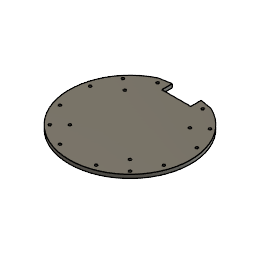
bot (Autodesk Fusion 360 design; units mm, degrees)
Autodesk Fusion 360 part; units mm, degrees
sketch "Esboço1" plane through (0, 0, 0) normal (0, 1, 0) x (1, 0, 0)
  circle A0 centre (0, 0) radius 90
  dimension "d1" = 180
  constraint coincident A0.centre origin
  measures "d1" diameter of A0
sketch "Esboço2" plane through (0, 0, 0) normal (0, 1, 0) x (1, 0, 0)
  circle A0 centre (0, 0) radius 80
  line L0 (0, 0) -> (0, 80)
  line L1 (0, 0) -> (0, -80)
  line L2 (0, 0) -> (80, 0)
  line L3 (0, 0) -> (-80, 0)
  line L4 (0, 0) -> (61.2836, 51.423)
  line L5 (0, 0) -> (80, 0) construction
  line L6 (0, 0) -> (-61.2836, 51.423)
  line L7 (0, 0) -> (80, 0) construction
  line L8 (0, 0) -> (-56.5685, -56.5685)
  line L9 (0, 0) -> (80, 0) construction
  line L10 (0, 0) -> (56.5685, -56.5685)
  line L11 (0, 0) -> (80, 0) construction
  dimension "d2" = 160
  dimension "d3" = 40
  dimension "d4" = 80
  dimension "d5" = 140
  dimension "d6" = 80
  dimension "d7" = 135
  dimension "d8" = 80
  dimension "d9" = 45
  constraint coincident A0.centre L0.start
  constraint coincident A0 L0.end
  constraint vertical L0
  constraint coincident A0 L1.end
  constraint parallel L0 L1
  constraint coincident A0 L2.end
  constraint perpendicular L0 L2
  constraint coincident A0 L3.end
  constraint perpendicular L1 L3
  constraint horizontal L5
  constraint horizontal L7
  constraint horizontal L9
  constraint horizontal L11
  measures "d2" diameter of A0
  measures "d3" angle of L4 L5
  measures "d4" distance of A0.centre L4.end
  measures "d5" angle of L6 L7
  measures "d6" distance of A0.centre L6.end
  measures "d7" angle of L8 L9
  measures "d8" distance of A0.centre L8.end
  measures "d9" angle of L10 L11
sketch "Esboço10" plane through (0, 4, 0) normal (0, 1, 0) x (-1, 0, 0)
  circle A0 centre (0, 0) radius 90
  circle A1 centre (0, 0) radius 80
  dimension "d156" = 160
  constraint coincident A0.centre A1.centre
  measures "d156" diameter of A1
sketch "Esboço11" plane through (0, 4, 0) normal (0, 1, 0) x (-1, 0, 0)
  line L0 (0, 0) -> (0, 89.7923) construction
  line L1 (0, 0) -> (0, -90.4079) construction
  line L2 (0, 0) -> (-89.4844, 0) construction
  line L3 (-89.4844, 0) -> (0, 0) construction
  line L4 (90.1162, 0) -> (0, 0) construction
  line L5 (0, 0) -> (-68.2901, -57.3022) construction
  line L6 (0, 0) -> (180, 0) construction
  line L7 (0, 0) -> (68.944, -57.8509) construction
  line L8 (0, 0) -> (90, 0) construction
  line L9 (0, 0) -> (-63.6396, 63.6396) construction
  line L10 (0, 0) -> (90, 0) construction
  line L11 (0, 0) -> (63.6396, 63.6396) construction
  line L12 (0, 0) -> (90, 0) construction
  dimension "d157" = 140
  dimension "d159" = 40
  dimension "d161" = 135
  dimension "d164" = 45
  constraint coincident L0.start L1.start
  constraint vertical L0
  constraint parallel L0 L1
  constraint perpendicular L0 L2
  constraint perpendicular L1 L4
  constraint horizontal L6
  constraint horizontal L8
  constraint horizontal L10
  constraint horizontal L12
  measures "d157" angle of L5 L6
  measures "d159" angle of L7 L8
  measures "d161" angle of L9 L10
  measures "d164" angle of L11 L12
sketch "Esboço13" plane through (0, 4, 0) normal (0, 1, 0) x (-1, 0, 0)
  line L0 (0, 0) -> (68.944, -57.8509) construction
  line L1 (0, 0) -> (90, 0) construction
  line L2 (68.944, -57.8509) -> (49.7929, -41.7812) construction
  line L3 (62.6595, 0) -> (-0.1598, -74.8652) construction
  line L4 (38.3771, -28.9387) -> (52.197, -12.4687)
  line L5 (35.1632, -32.7689) -> (21.3439, -49.2381)
  line L6 (20.2359, -54.8368) -> (24.0661, -58.0507)
  line L7 (32.9399, -27.6399) -> (34.5469, -25.7248)
  line L8 (32.9399, -27.6399) -> (31.3329, -29.555)
  line L9 (31.3329, -29.555) -> (35.1632, -32.7689)
  line L10 (34.5469, -25.7248) -> (38.3771, -28.9387)
  circle A0 centre (34.855, -29.2468) radius 1.35
  line L11 (50.2508, -38.9019) -> (47.0369, -42.7321)
  line L12 (47.0369, -42.7321) -> (43.2066, -39.5182)
  line L13 (50.2508, -38.9019) -> (46.4206, -35.688)
  circle A1 centre (46.7287, -39.21) radius 1.35
  line L14 (59.4327, -12.0132) -> (57.8257, -13.9283) construction
  circle A2 centre (57.8257, -13.9283) radius 1.35
  line L15 (22.151, -56.4437) -> (23.758, -54.5286) construction
  circle A3 centre (23.758, -54.5286) radius 1.35
  circle A4 centre (0, 0) radius 65 construction
  line L16 (0, 0) -> (0, -90.5075) construction
  line L17 (55.9131, -12.3183) -> (57.5176, -10.4062)
  line L18 (59.7408, -15.5352) -> (61.3478, -13.6201)
  line L19 (55.9131, -12.3183) -> (54.3037, -14.2364)
  line L20 (54.3037, -14.2364) -> (52.197, -12.4687)
  line L21 (58.1339, -17.4503) -> (60.2406, -19.2179)
  line L22 (59.7408, -15.5352) -> (58.1339, -17.4503)
  line L23 (61.3478, -13.6201) -> (57.5176, -10.4062)
  line L24 (27.2801, -54.2205) -> (29.3867, -55.9881)
  line L25 (23.4505, -51.0058) -> (20.2359, -54.8368)
  line L26 (20.2359, -54.8368) -> (24.0661, -58.0507)
  line L27 (24.0661, -58.0507) -> (27.2801, -54.2205)
  line L28 (23.4505, -51.0058) -> (21.3439, -49.2381)
  line L29 (29.3867, -55.9881) -> (43.2066, -39.5182)
  line L30 (46.4206, -35.688) -> (60.2406, -19.2179)
  circle A5 centre (0, 0) radius 53.25 construction
  circle A6 centre (40.7919, -34.2284) radius 7.75 construction
  circle A7 centre (40.7919, -34.2284) radius 26.5 construction
  line L31 (22.151, -56.4437) -> (59.4327, -12.0132) construction
  line L32 (0, 0) -> (0, -90.4079)
  line L33 (-20.2359, -54.8368) -> (-24.0661, -58.0507)
  circle A8 centre (-23.758, -54.5286) radius 1.35
  line L34 (-35.1632, -32.7689) -> (-21.3439, -49.2381)
  line L35 (-31.3329, -29.555) -> (-35.1632, -32.7689)
  line L36 (-32.9399, -27.6399) -> (-31.3329, -29.555)
  line L37 (-32.9399, -27.6399) -> (-34.5469, -25.7248)
  line L38 (-34.5469, -25.7248) -> (-38.3771, -28.9387)
  line L39 (-38.3771, -28.9387) -> (-52.197, -12.4687)
  line L40 (-54.3037, -14.2364) -> (-52.197, -12.4687)
  line L41 (-55.9131, -12.3183) -> (-54.3037, -14.2364)
  line L42 (-55.9131, -12.3183) -> (-57.5176, -10.4062)
  line L43 (-61.3478, -13.6201) -> (-57.5176, -10.4062)
  line L44 (-59.7408, -15.5352) -> (-61.3478, -13.6201)
  line L45 (-59.7408, -15.5352) -> (-58.1339, -17.4503)
  line L46 (-58.1339, -17.4503) -> (-60.2406, -19.2179)
  line L47 (-46.4206, -35.688) -> (-60.2406, -19.2179)
  line L48 (-50.2508, -38.9019) -> (-46.4206, -35.688)
  line L49 (-50.2508, -38.9019) -> (-47.0369, -42.7321)
  line L50 (-47.0369, -42.7321) -> (-43.2066, -39.5182)
  line L51 (-29.3867, -55.9881) -> (-43.2066, -39.5182)
  line L52 (-27.2801, -54.2205) -> (-29.3867, -55.9881)
  line L53 (-23.4505, -51.0058) -> (-21.3439, -49.2381)
  circle A9 centre (-46.7287, -39.21) radius 1.35
  circle A10 centre (-34.855, -29.2468) radius 1.35
  circle A11 centre (-57.8257, -13.9283) radius 1.35
  line L54 (-24.0661, -58.0507) -> (-27.2801, -54.2205)
  line L55 (-23.4505, -51.0058) -> (-20.2359, -54.8368)
  line L56 (50.2508, -38.9019) -> (47.0369, -42.7321)
  line L57 (47.0369, -42.7321) -> (43.2066, -39.5182)
  circle A12 centre (46.7287, -39.21) radius 1.35
  line L58 (50.2508, -38.9019) -> (46.4206, -35.688)
  line L59 (46.4206, -35.688) -> (60.2406, -19.2179)
  line L60 (59.7408, -15.5352) -> (58.1339, -17.4503)
  circle A13 centre (57.8257, -13.9283) radius 1.35
  line L61 (58.1339, -17.4503) -> (60.2406, -19.2179)
  line L62 (59.7408, -15.5352) -> (61.3478, -13.6201)
  line L63 (61.3478, -13.6201) -> (57.5176, -10.4062)
  line L64 (55.9131, -12.3183) -> (54.3037, -14.2364)
  line L65 (55.9131, -12.3183) -> (57.5176, -10.4062)
  line L66 (54.3037, -14.2364) -> (52.197, -12.4687)
  line L67 (38.3771, -28.9387) -> (52.197, -12.4687)
  line L68 (34.5469, -25.7248) -> (38.3771, -28.9387)
  circle A14 centre (34.855, -29.2468) radius 1.35
  line L69 (31.3329, -29.555) -> (35.1632, -32.7689)
  line L70 (32.9399, -27.6399) -> (34.5469, -25.7248)
  line L71 (32.9399, -27.6399) -> (31.3329, -29.555)
  line L72 (35.1632, -32.7689) -> (21.3439, -49.2381)
  line L73 (29.3867, -55.9881) -> (43.2066, -39.5182)
  line L74 (27.2801, -54.2205) -> (29.3867, -55.9881)
  line L75 (24.0661, -58.0507) -> (27.2801, -54.2205)
  line L76 (20.2359, -54.8368) -> (24.0661, -58.0507)
  circle A15 centre (23.758, -54.5286) radius 1.35
  line L77 (23.4505, -51.0058) -> (20.2359, -54.8368)
  line L78 (23.4505, -51.0058) -> (21.3439, -49.2381)
  line L79 (0, 0) -> (63.6396, 63.6396) construction
  line L80 (0, 0) -> (90, 0) construction
  line L81 (63.6396, 63.6396) -> (33.9411, 33.9411) construction
  line L82 (33.9411, 33.9411) -> (0, 67.8823) construction
  line L83 (33.9411, 33.9411) -> (67.8823, 0) construction
  line L84 (0, 0) -> (0, 90) construction
  line L85 (0, 0) -> (-89.8338, 0) construction
  line L86 (41.7925, 40.6545) -> (26.5896, 55.8573)
  line L87 (24.6452, 53.9127) -> (26.5896, 55.8573)
  line L88 (22.8773, 55.6805) -> (24.6452, 53.9127)
  line L89 (22.8773, 55.6805) -> (21.1096, 57.4483)
  line L90 (21.1096, 57.4483) -> (17.5741, 53.9127)
  line L91 (19.3391, 52.1477) -> (17.5741, 53.9127)
  line L92 (19.3391, 52.1477) -> (21.1096, 50.3772)
  circle A16 centre (21.1096, 53.9127) radius 1.35
  line L93 (21.1096, 50.3772) -> (19.1651, 48.4327)
  line L94 (34.3679, 33.2299) -> (19.1651, 48.4327)
  line L95 (30.8323, 29.6943) -> (34.3679, 33.2299)
  circle A17 centre (34.3679, 29.6943) radius 1.35
  line L96 (32.6001, 27.9266) -> (30.8323, 29.6943)
  line L97 (32.6001, 27.9266) -> (34.3679, 26.1588)
  line L98 (34.3679, 26.1588) -> (37.9034, 29.6943)
  line L99 (37.9034, 29.6943) -> (53.1055, 14.4923)
  line L100 (45.328, 44.19) -> (41.7925, 40.6545)
  line L101 (45.328, 44.19) -> (48.8636, 40.6545)
  line L102 (48.8636, 40.6545) -> (45.328, 37.119)
  circle A18 centre (45.328, 40.6545) radius 1.35
  line L103 (60.5308, 21.9162) -> (45.328, 37.119)
  line L104 (62.1218, 16.4361) -> (58.5863, 19.9716)
  line L105 (58.5863, 19.9716) -> (60.5308, 21.9162)
  line L106 (55.05, 16.4368) -> (58.5863, 12.9005)
  line L107 (55.05, 16.4368) -> (53.1055, 14.4923)
  line L108 (58.5863, 12.9005) -> (62.1218, 16.4361)
  circle A19 centre (58.5863, 16.4361) radius 1.35
  line L109 (-58.5863, 12.9005) -> (-62.1218, 16.4361)
  line L110 (-55.05, 16.4368) -> (-58.5863, 12.9005)
  circle A20 centre (-58.5863, 16.4361) radius 1.35
  line L111 (-62.1218, 16.4361) -> (-58.5863, 19.9716)
  line L112 (-58.5863, 19.9716) -> (-60.5308, 21.9162)
  line L113 (-55.05, 16.4368) -> (-53.1055, 14.4923)
  line L114 (-37.9034, 29.6943) -> (-53.1055, 14.4923)
  line L115 (-60.5308, 21.9162) -> (-45.328, 37.119)
  line L116 (-48.8636, 40.6545) -> (-45.328, 37.119)
  line L117 (-45.328, 44.19) -> (-48.8636, 40.6545)
  circle A21 centre (-45.328, 40.6545) radius 1.35
  line L118 (-45.328, 44.19) -> (-41.7925, 40.6545)
  line L119 (-41.7925, 40.6545) -> (-26.5896, 55.8573)
  line L120 (-34.3679, 26.1588) -> (-37.9034, 29.6943)
  line L121 (-32.6001, 27.9266) -> (-34.3679, 26.1588)
  line L122 (-32.6001, 27.9266) -> (-30.8323, 29.6943)
  circle A22 centre (-34.3679, 29.6943) radius 1.35
  line L123 (-30.8323, 29.6943) -> (-34.3679, 33.2299)
  line L124 (-34.3679, 33.2299) -> (-19.1651, 48.4327)
  line L125 (-24.6452, 53.9127) -> (-26.5896, 55.8573)
  line L126 (-22.8773, 55.6805) -> (-24.6452, 53.9127)
  line L127 (-22.8773, 55.6805) -> (-21.1096, 57.4483)
  circle A23 centre (-21.1096, 53.9127) radius 1.35
  line L128 (-21.1096, 57.4483) -> (-17.5741, 53.9127)
  line L129 (-19.3391, 52.1477) -> (-17.5741, 53.9127)
  line L130 (-19.3391, 52.1477) -> (-21.1096, 50.3772)
  line L131 (-21.1096, 50.3772) -> (-19.1651, 48.4327)
  line L132 (0, -65) -> (15, -65)
  line L133 (0, -65) -> (-15, -65)
  line L134 (-15, -65) -> (-15, -55)
  line L135 (-15, -55) -> (15, -55)
  line L136 (15, -55) -> (15, -65)
  line L137 (15, -65) -> (15, -80)
  line L138 (15, -80) -> (-15, -80)
  line L139 (-15, -80) -> (-15, -65)
  dimension "d166" = 40
  dimension "d167" = 25
  dimension "d176" = 2.5
  dimension "d177" = 2.5
  dimension "d178" = 5
  dimension "d179" = 2.7
  dimension "d182" = 5
  dimension "d183" = 2.7
  dimension "d186" = 2.7
  dimension "d187" = 2.5
  dimension "d188" = 2.7
  dimension "d194" = 5
  dimension "d195" = 2.5
  dimension "d196" = 2.75
  dimension "d197" = 2.75
  dimension "d199" = 13.5118
  dimension "d200" = 15.0096
  dimension "d201" = 21.5
  dimension "d202" = 21.499
  dimension "d203" = 2.5
  dimension "d204" = 2.5
  dimension "d205" = 2.5
  dimension "d206" = 2.5
  dimension "d207" = 5
  dimension "d208" = 2.75
  dimension "d209" = 2.75
  dimension "d210" = 5
  dimension "d211" = 5
  dimension "d212" = 5
  dimension "d215" = 29
  dimension "d216" = 24.1299
  dimension "d217" = 24.1299
  dimension "d218" = 2.5
  dimension "d220" = 2.5
  dimension "d222" = 2.5
  dimension "d223" = 2.5
  dimension "d224" = 2.5
  dimension "d225" = 5
  dimension "d226" = 2.7
  dimension "d227" = 5
  dimension "d228" = 2.7
  dimension "d229" = 2.7
  dimension "d230" = 2.7
  dimension "d231" = 5
  dimension "d232" = 2.5
  dimension "d233" = 2.75
  dimension "d234" = 2.75
  dimension "d235" = 21.5
  dimension "d236" = 21.499
  dimension "d237" = 2.5
  dimension "d238" = 2.5
  dimension "d239" = 2.5
  dimension "d240" = 2.5
  dimension "d241" = 5
  dimension "d242" = 2.75
  dimension "d243" = 2.75
  dimension "d244" = 5
  dimension "d245" = 5
  dimension "d246" = 5
  dimension "d247" = 2.5
  dimension "d248" = 2.5
  dimension "d249" = 45
  dimension "d250" = 90
  dimension "d251" = 42
  dimension "d252" = 90
  dimension "d253" = 5
  dimension "d254" = 2.7
  dimension "d255" = 5
  dimension "d256" = 2.7
  dimension "d257" = 2.7
  dimension "d258" = 5
  dimension "d259" = 2.75
  dimension "d260" = 2.75
  dimension "d261" = 21.5
  dimension "d262" = 21.499
  dimension "d263" = 2.5
  dimension "d264" = 2.5
  dimension "d265" = 5
  dimension "d266" = 2.75
  dimension "d267" = 5
  dimension "d268" = 5
  dimension "d269" = 2.5
  dimension "d270" = 2.5
  dimension "d271" = 2.5
  dimension "d272" = 2.7
  dimension "d273" = 21.499
  dimension "d274" = 2.75
  dimension "d275" = 2.5
  dimension "d283" = 15
  dimension "d284" = 15
  dimension "d285" = 10
  dimension "d286" = 30
  dimension "d287" = 15
  dimension "d288" = 30
  constraint horizontal L1
  constraint coincident L0.start L1.start
  constraint parallel L0 L2
  constraint coincident L1 L3.start
  constraint perpendicular L0 L3
  constraint perpendicular L0 L4
  constraint perpendicular L3 L6
  constraint perpendicular L0 L7
  constraint perpendicular L0 L8
  constraint coincident L3 L5.start
  constraint perpendicular L8 L9
  constraint perpendicular L4 L10
  constraint coincident L14.end A2.centre
  constraint perpendicular L6 L15
  constraint coincident L15.end A3.centre
  constraint coincident L2.end A4
  constraint vertical L16
  constraint perpendicular L21 L22
  constraint parallel L17 L19
  constraint parallel L3 L19
  constraint coincident L3 L5.end
  constraint perpendicular L6 L25
  constraint perpendicular L15 L26
  constraint perpendicular L24 L27
  constraint coincident L6 L15.start
  constraint collinear L29 L30
  constraint perpendicular L11 L12
  constraint coincident L0 A6.centre
  constraint coincident A5 A6.centre
  constraint coincident A0.centre A6
  constraint concentric A6 A7
  constraint coincident L15.end A7
  constraint parallel L6 L28
  constraint parallel L24 L26
  constraint perpendicular L23 L31
  constraint parallel L25 L31
  constraint parallel L11 L31
  constraint perpendicular L13 L30
  constraint perpendicular L12 L29
  constraint perpendicular L19 L20
  constraint symmetric L7.start L32 L36.start
  constraint symmetric L7.end L32 L37.end
  constraint symmetric L8.end L32 L35.start
  constraint symmetric L5.start L32 L34.start
  constraint symmetric L4.start L32 L38.end
  constraint symmetric A0 L32 A10
  constraint symmetric L11.start L32 L48.start
  constraint symmetric L11.end L32 L49.end
  constraint symmetric L12.end L32 L50.end
  constraint symmetric L13.end L32 L47.start
  constraint symmetric A1 L32 A9
  constraint symmetric A2 L32 A11
  constraint symmetric A3 L32 A8
  constraint symmetric L18.start L32 L44.start
  constraint symmetric L17.start L32 L41.start
  constraint symmetric L17.end L32 L42.end
  constraint symmetric L18.end L32 L43.start
  constraint symmetric L19.end L32 L40.start
  constraint symmetric L4.end L32 L39.end
  constraint symmetric L21.end L32 L46.end
  constraint symmetric L21.start L32 L45.end
  constraint symmetric L5.end L32 L34.end
  constraint symmetric L24.end L32 L51.start
  constraint symmetric L25.start L32 L53.start
  constraint symmetric L6.start L32 L33.start
  constraint symmetric L6.end L32 L33.end
  constraint symmetric L24.start L32 L52.start
  constraint perpendicular L69 L71
  constraint perpendicular L67 L68
  constraint perpendicular L60 L61
  constraint parallel L64 L65
  constraint perpendicular L76 L77
  constraint perpendicular L74 L75
  constraint collinear L59 L73
  constraint perpendicular L56 L57
  constraint parallel L76 L78
  constraint perpendicular L58 L59
  constraint perpendicular L57 L73
  constraint perpendicular L64 L66
  constraint horizontal L80
  constraint parallel L79 L81
  constraint perpendicular L79 L82
  constraint coincident L1 L83.end
  constraint perpendicular L81 L83
  constraint vertical L84
  constraint coincident L84 L82.end
  constraint parallel L1 L85
  constraint perpendicular L94 L95
  constraint perpendicular L87 L88
  constraint perpendicular L106 L108
  constraint perpendicular L104 L105
  constraint parallel L107 L108
  constraint perpendicular L92 L93
  constraint symmetric L84 L91.start L129.start
  constraint symmetric L84 L89.end L127.end
  constraint symmetric L84 L93.end L124.end
  constraint symmetric L84 L86.end L119.end
  constraint symmetric L84 L88.start L126.start
  constraint symmetric L84 L92.end L130.end
  constraint symmetric L84 L97.end L120.start
  constraint symmetric L84 L99.end L113.end
  constraint symmetric L84 L95.start L122.end
  constraint symmetric L84 L98.end L114.start
  constraint symmetric L84 L94.start L123.end
  constraint symmetric L84 L90.end L128.end
  constraint symmetric L84 L101.end L116.start
  constraint symmetric L84 L100.start L117.start
  constraint symmetric L84 L102.end L115.end
  constraint symmetric L84 L86.start L118.end
  constraint symmetric L84 L104.start L109.end
  constraint symmetric L84 L87.start L125.start
  constraint symmetric L84 L104.end L111.end
  constraint symmetric L84 L103.start L112.end
  constraint symmetric L84 L106.start L110.start
  constraint symmetric L84 L106.end L109.start
  constraint symmetric L84 L96.start L121.start
  constraint symmetric L84 A16 A23
  constraint symmetric L84 A17 A22
  constraint symmetric L84 A18 A21
  constraint symmetric L84 A19 A20
  constraint coincident L32 L132.start
  constraint coincident A4 L132.start
  constraint perpendicular L32 L132
  constraint perpendicular L16 L133
  constraint perpendicular L133 L134
  constraint perpendicular L134 L135
  constraint perpendicular L132 L137
  constraint perpendicular L32 L138
  measures "d166" angle of L0 L1
  measures "d167" distance of L0.end L2.end
  measures "d176" distance of L7.start L7.end
  measures "d177" distance of L7.start L8.end
  measures "d178" distance of L7.end L4.start
  measures "d179" diameter of A0
  measures "d182" distance of L11.start L11.end
  measures "d183" diameter of A1
  measures "d186" diameter of A2
  measures "d187" distance of L15.start L15.end
  measures "d188" diameter of A3
  measures "d194" distance of L6.start L6.end
  measures "d195" distance of L15.end L25
  measures "d196" distance of L5.end L25.start
  measures "d197" distance of L24.end L24.start
  measures "d199" horizontal distance of L24.start A6.centre
  measures "d200" vertical distance of L5.end A6.centre
  measures "d201" distance of L12.end L24.end
  measures "d202" distance of L5.start L5.end
  measures "d203" distance of L7.start A0.centre
  measures "d204" distance of L9 A0.centre
  measures "d205" distance of L12 A1.centre
  measures "d206" distance of L11 A1.centre
  measures "d207" distance of L11.start L13.end
  measures "d208" distance of L21.end L21.start
  measures "d209" distance of L19.end L4.end
  measures "d210" distance of L17.end L19.end
  measures "d211" distance of L17.end L18.end
  measures "d212" distance of L18.end L21.start
  measures "d215" distance of L14.start A6.centre
  measures "d216" distance of L19.end A6.centre
  measures "d217" distance of L21.start A6.centre
  measures "d218" distance of L14.start L14.end
  measures "d220" distance of L18.start L18.end
  measures "d222" distance of L14.end L19
  measures "d223" distance of L7.start L7.end
  measures "d224" distance of L7.start L8.end
  measures "d225" distance of L7.end L4.start
  measures "d226" diameter of A14
  measures "d227" distance of L11.end L11.start
  measures "d228" diameter of A12
  measures "d229" diameter of A13
  measures "d230" diameter of A15
  measures "d231" distance of L6.end L6.start
  measures "d232" distance of L15.end L77
  measures "d233" distance of L5.end L25.start
  measures "d234" distance of L24.start L24.end
  measures "d235" distance of L12.end L24.end
  measures "d236" distance of L5.end L5.start
  measures "d237" distance of L7.start A0.centre
  measures "d238" distance of A0.centre L69
  measures "d239" distance of A1.centre L57
  measures "d240" distance of A1.centre L56
  measures "d241" distance of L11.start L13.end
  measures "d242" distance of L21.start L21.end
  measures "d243" distance of L4.end L19.end
  measures "d244" distance of L17.end L19.end
  measures "d245" distance of L17.end L18.end
  measures "d246" distance of L21.start L18.end
  measures "d247" distance of L18.start L18.end
  measures "d248" distance of L14.end L64
  measures "d249" angle of L79 L80
  measures "d250" distance of L0.start L79.end
  measures "d251" distance of L79.end L81.end
  measures "d252" distance of L0.start L84.end
  measures "d253" distance of L95.start L94.start
  measures "d254" diameter of A17
  measures "d255" distance of L101.end L100.start
  measures "d256" diameter of A18
  measures "d257" diameter of A16
  measures "d258" distance of L104.start L106.end
  measures "d259" distance of L99.end L106.start
  measures "d260" distance of L104.end L103.start
  measures "d261" distance of L102.end L103.start
  measures "d262" distance of L99.end L98.end
  measures "d263" distance of A17.centre L98
  measures "d264" distance of A18.centre L101
  measures "d265" distance of L100.start L86.start
  measures "d266" distance of L87.start L86.end
  measures "d267" distance of L90.end L89.end
  measures "d268" distance of L87.start L89.end
  measures "d269" distance of L88.start L89.end
  measures "d270" distance of L96.start L95.start
  measures "d271" distance of L96.start L97.end
  measures "d272" diameter of A19
  measures "d273" distance of L99.end L98.end
  measures "d274" distance of L93.end L92.end
  measures "d275" distance of L89.end L88.start
  measures "d283" distance of L132.start L132.end
  measures "d284" distance of L132.start L133.end
  measures "d285" distance of L133.end L134.end
  measures "d286" distance of L134.end L135.end
  measures "d287" distance of L132.end L137.end
  measures "d288" distance of L137.end L138.end
sketch "Esboço14" plane through (0, 4, 0) normal (0, 1, 0) x (-1, 0, 0)
  circle A0 centre (0, 0) radius 90
  circle A1 centre (0, 0) radius 67.5
  dimension "d276" = 135
  constraint coincident A0.centre A1.centre
  measures "d276" diameter of A1
sketch "Esboço15" plane through (0, 0, 0) normal (0, 1, 0) x (1, 0, 0)
  line L0 (0, 0) -> (0, 92.4179) construction
  line L1 (0, 0) -> (93.6244, 0) construction
  line L2 (0, 0) -> (0, -88.0745) construction
  line L3 (0, 0) -> (-79.8703, 0) construction
  line L4 (0, 0) -> (88.3333, 0) construction
  line L5 (0, 0) -> (-68.7403, 57.6799) construction
  line L6 (0, 0) -> (89.7341, 0) construction
  line L7 (0, 0) -> (60.1115, -60.1115) construction
  line L8 (0, 0) -> (85.0106, 0) construction
  line L9 (0, 0) -> (-55.023, -55.023) construction
  line L10 (0, 0) -> (77.8143, 0) construction
  line L11 (0, 0) -> (-42.1324, 35.3533) construction
  line L12 (0, 0) -> (-38.8909, -38.8909) construction
  line L13 (-42.1324, 35.3533) -> (-35.7046, 43.0138) construction
  line L14 (-42.1324, 35.3533) -> (-48.5603, 27.6929) construction
  line L15 (-38.8909, -38.8909) -> (-45.9619, -31.8198) construction
  line L16 (-38.8909, -38.8909) -> (-31.8198, -45.9619) construction
  line L17 (-36.2801, 33.7714) -> (-22.428, 50.2797)
  line L18 (-53.4104, 13.3563) -> (-39.5583, 29.8646)
  line L19 (-50.3291, 42.2311) -> (-48.69, 44.1846)
  line L20 (-50.3291, 42.2311) -> (-51.9682, 40.2777)
  line L21 (-51.9682, 40.2777) -> (-48.0614, 36.9995)
  line L22 (-48.69, 44.1846) -> (-44.7832, 40.9063)
  line L23 (-30.9311, 57.4146) -> (-44.7832, 40.9063)
  line L24 (-48.0614, 36.9995) -> (-61.9135, 20.4913)
  line L25 (-23.4013, 57.754) -> (-21.4479, 56.1148)
  line L26 (-23.4013, 57.754) -> (-25.3548, 59.3931)
  line L27 (-21.4479, 56.1148) -> (-24.7262, 52.208)
  line L28 (-25.3548, 59.3931) -> (-28.633, 55.4862)
  line L29 (-22.428, 50.2797) -> (-24.7262, 52.208)
  line L30 (-28.633, 55.4862) -> (-30.9311, 57.4146)
  line L31 (-60.9401, 13.017) -> (-62.8936, 14.6561)
  line L32 (-60.9401, 13.017) -> (-58.9867, 11.3779)
  line L33 (-58.9867, 11.3779) -> (-55.7085, 15.2847)
  line L34 (-62.8936, 14.6561) -> (-59.6153, 18.5629)
  line L35 (-61.9135, 20.4913) -> (-59.6153, 18.5629)
  line L36 (-55.7085, 15.2847) -> (-53.4104, 13.3563)
  line L37 (-60.9401, 13.017) -> (-23.4013, 57.754) construction
  line L38 (-39.5583, 29.8646) -> (-36.0345, 26.9078)
  line L39 (-36.2801, 33.7714) -> (-32.7563, 30.8146)
  line L40 (-36.0345, 26.9078) -> (-32.7563, 30.8146)
  line L41 (-36.7696, -33.1633) -> (-52.0077, -17.9252)
  line L42 (-33.1633, -36.7696) -> (-17.9252, -52.0077)
  line L43 (-31.7137, -31.7137) -> (-29.9106, -33.5169)
  line L44 (-31.7137, -31.7137) -> (-33.5169, -29.9106)
  line L45 (-29.9106, -33.5169) -> (-33.1633, -36.7696)
  line L46 (-33.5169, -29.9106) -> (-36.7696, -33.1633)
  line L47 (-18.2434, -59.5384) -> (-16.4402, -57.7353)
  line L48 (-18.2434, -59.5384) -> (-20.0465, -61.3415)
  line L49 (-20.0465, -61.3415) -> (-23.6527, -57.7353)
  line L50 (-16.4402, -57.7353) -> (-20.0465, -54.129)
  line L51 (-59.5384, -18.2434) -> (-57.7353, -16.4402)
  line L52 (-59.5384, -18.2434) -> (-61.3415, -20.0465)
  line L53 (-61.3415, -20.0465) -> (-57.7353, -23.6527)
  line L54 (-57.7353, -16.4402) -> (-54.129, -20.0465)
  line L55 (-46.4216, -46.4216) -> (-44.6184, -48.2247)
  line L56 (-46.4216, -46.4216) -> (-48.2247, -44.6184)
  line L57 (-48.2247, -44.6184) -> (-44.6184, -41.0122)
  line L58 (-44.6184, -48.2247) -> (-41.0122, -44.6184)
  line L59 (-59.8566, -25.774) -> (-57.7353, -23.6527)
  line L60 (-54.129, -20.0465) -> (-52.0077, -17.9252)
  line L61 (-25.774, -59.8566) -> (-41.0122, -44.6184)
  line L62 (-44.6184, -41.0122) -> (-59.8566, -25.774)
  line L63 (-17.9252, -52.0077) -> (-20.0465, -54.129)
  line L64 (-23.6527, -57.7353) -> (-25.774, -59.8566)
  circle A0 centre (-57.6999, -20.0818) radius 1.4
  circle A1 centre (-33.3754, -33.3754) radius 1.4
  circle A2 centre (-44.5831, -44.5831) radius 1.4
  circle A3 centre (-20.0818, -57.6999) radius 1.4
  circle A4 centre (-36.1956, 30.3717) radius 1.4
  circle A5 centre (-48.3374, 40.5599) radius 1.4
  circle A6 centre (-25.0726, 55.7622) radius 1.4
  circle A7 centre (-59.2689, 15.0087) radius 1.4
  line L65 (50.3291, 42.2311) -> (51.9682, 40.2777)
  circle A8 centre (48.3374, 40.5599) radius 1.4
  line L66 (28.633, 55.4862) -> (30.9311, 57.4146)
  line L67 (25.3548, 59.3931) -> (28.633, 55.4862)
  line L68 (42.1324, 35.3533) -> (35.7046, 43.0138) construction
  line L69 (58.9867, 11.3779) -> (55.7085, 15.2847)
  line L70 (60.9401, 13.017) -> (62.8936, 14.6561)
  line L71 (55.7085, 15.2847) -> (53.4104, 13.3563)
  line L72 (53.4104, 13.3563) -> (39.5583, 29.8646)
  line L73 (39.5583, 29.8646) -> (36.0345, 26.9078)
  line L74 (62.8936, 14.6561) -> (59.6153, 18.5629)
  line L75 (22.428, 50.2797) -> (24.7262, 52.208)
  line L76 (23.4013, 57.754) -> (21.4479, 56.1148)
  line L77 (50.3291, 42.2311) -> (48.69, 44.1846)
  line L78 (60.9401, 13.017) -> (23.4013, 57.754) construction
  line L79 (21.4479, 56.1148) -> (24.7262, 52.208)
  line L80 (42.1324, 35.3533) -> (48.5603, 27.6929) construction
  line L81 (36.0345, 26.9078) -> (32.7563, 30.8146)
  line L82 (36.2801, 33.7714) -> (22.428, 50.2797)
  line L83 (60.9401, 13.017) -> (58.9867, 11.3779)
  circle A9 centre (59.2689, 15.0087) radius 1.4
  line L84 (30.9311, 57.4146) -> (44.7832, 40.9063)
  line L85 (48.0614, 36.9995) -> (61.9135, 20.4913)
  line L86 (48.69, 44.1846) -> (44.7832, 40.9063)
  line L87 (61.9135, 20.4913) -> (59.6153, 18.5629)
  line L88 (23.4013, 57.754) -> (25.3548, 59.3931)
  line L89 (51.9682, 40.2777) -> (48.0614, 36.9995)
  circle A10 centre (36.1956, 30.3717) radius 1.4
  circle A11 centre (25.0726, 55.7622) radius 1.4
  line L90 (36.2801, 33.7714) -> (32.7563, 30.8146)
  line L91 (18.2434, -59.5384) -> (20.0465, -61.3415)
  line L92 (16.4402, -57.7353) -> (20.0465, -54.129)
  line L93 (23.6527, -57.7353) -> (25.774, -59.8566)
  line L94 (17.9252, -52.0077) -> (20.0465, -54.129)
  line L95 (54.129, -20.0465) -> (52.0077, -17.9252)
  line L96 (48.2247, -44.6184) -> (44.6184, -41.0122)
  circle A12 centre (57.6999, -20.0818) radius 1.4
  line L97 (44.6184, -48.2247) -> (41.0122, -44.6184)
  line L98 (61.3415, -20.0465) -> (57.7353, -23.6527)
  line L99 (38.8909, -38.8909) -> (31.8198, -45.9619) construction
  line L100 (59.5384, -18.2434) -> (61.3415, -20.0465)
  line L101 (57.7353, -16.4402) -> (54.129, -20.0465)
  line L102 (31.7137, -31.7137) -> (29.9106, -33.5169)
  line L103 (31.7137, -31.7137) -> (33.5169, -29.9106)
  line L104 (38.8909, -38.8909) -> (45.9619, -31.8198) construction
  circle A13 centre (33.3754, -33.3754) radius 1.4
  line L105 (46.4216, -46.4216) -> (44.6184, -48.2247)
  line L106 (59.8566, -25.774) -> (57.7353, -23.6527)
  line L107 (0, 0) -> (38.8909, -38.8909) construction
  line L108 (46.4216, -46.4216) -> (48.2247, -44.6184)
  circle A14 centre (44.5831, -44.5831) radius 1.4
  line L109 (20.0465, -61.3415) -> (23.6527, -57.7353)
  circle A15 centre (20.0818, -57.6999) radius 1.4
  line L110 (0, 0) -> (55.023, -55.023) construction
  line L111 (44.6184, -41.0122) -> (59.8566, -25.774)
  line L112 (59.5384, -18.2434) -> (57.7353, -16.4402)
  line L113 (25.774, -59.8566) -> (41.0122, -44.6184)
  line L114 (18.2434, -59.5384) -> (16.4402, -57.7353)
  line L115 (36.7696, -33.1633) -> (52.0077, -17.9252)
  line L116 (33.5169, -29.9106) -> (36.7696, -33.1633)
  line L117 (29.9106, -33.5169) -> (33.1633, -36.7696)
  line L118 (33.1633, -36.7696) -> (17.9252, -52.0077)
  point P0 (68.7403, 57.6799)
  dimension "d294" = 45
  dimension "d295" = 135
  dimension "d296" = 55
  dimension "d297" = 55
  dimension "d298" = 10
  dimension "d299" = 10
  dimension "d300" = 10
  dimension "d301" = 10
  dimension "d305" = 11.1
  dimension "d306" = 48.2
  dimension "d307" = 11.1
  dimension "d318" = 2.55
  dimension "d319" = 2.55
  dimension "d321" = 2.55
  dimension "d322" = 2.55
  dimension "d324" = 2.55
  dimension "d325" = 2.55
  dimension "d328" = 4.6
  dimension "d333" = 11.1
  dimension "d334" = 48.2
  dimension "d336" = 2.55
  dimension "d337" = 2.55
  dimension "d340" = 2.55
  dimension "d341" = 2.55
  dimension "d344" = 2.55
  dimension "d345" = 2.55
  dimension "d348" = 2.55
  dimension "d349" = 2.55
  dimension "d365" = 2.8
  dimension "d367" = 2.8
  dimension "d369" = 2.8
  dimension "d371" = 2.8
  dimension "d373" = 2.8
  dimension "d375" = 2.8
  dimension "d377" = 2.8
  dimension "d379" = 2.8
  constraint coincident L0.start L1.start
  constraint vertical L0
  constraint perpendicular L0 L1
  constraint perpendicular L1 L2
  constraint perpendicular L2 L3
  constraint horizontal L4
  constraint horizontal L6
  constraint horizontal L8
  constraint horizontal L10
  constraint parallel L5 L11
  constraint parallel L9 L12
  constraint perpendicular L5 L13
  constraint perpendicular L5 L14
  constraint perpendicular L9 L15
  constraint perpendicular L9 L16
  constraint perpendicular L5 L17
  constraint perpendicular L17 L29
  constraint perpendicular L5 L23
  constraint perpendicular L23 L35
  constraint perpendicular L5 L19
  constraint perpendicular L21 L23
  constraint perpendicular L22 L23
  constraint coincident L21.end L23
  constraint collinear L23 L24
  constraint perpendicular L27 L29
  constraint coincident L28.end L29
  constraint perpendicular L28 L29
  constraint collinear L29 L30
  constraint coincident L33.end L35
  constraint perpendicular L33 L35
  constraint perpendicular L34 L35
  constraint collinear L35 L36
  constraint perpendicular L25 L37
  constraint perpendicular L17 L39
  constraint perpendicular L39 L40
  constraint perpendicular L12 L41
  constraint perpendicular L12 L42
  constraint perpendicular L42 L63
  constraint perpendicular L9 L61
  constraint perpendicular L9 L43
  constraint perpendicular L12 L44
  constraint perpendicular L42 L45
  constraint perpendicular L41 L46
  constraint coincident L49.end L63
  constraint perpendicular L49 L63
  constraint perpendicular L50 L63
  constraint perpendicular L53 L59
  constraint perpendicular L54 L59
  constraint coincident L54.end L59
  constraint perpendicular L9 L55
  constraint coincident L57.end L61
  constraint perpendicular L57 L61
  constraint perpendicular L58 L61
  constraint collinear L59 L60
  constraint collinear L61 L62
  constraint collinear L63 L64
  constraint symmetric L0 L5.end P0
  constraint symmetric L0 L11.end L68.start
  constraint symmetric L0 L13.end L68.end
  constraint symmetric L0 L14.end L80.end
  constraint symmetric L0 L17.end L75.start
  constraint symmetric L0 L23.start L66.end
  constraint symmetric L0 L24.end L85.end
  constraint symmetric L0 L18.start L71.end
  constraint symmetric L0 L19.start L65.start
  constraint symmetric L0 L25.start L76.start
  constraint symmetric L0 L31.start L70.start
  constraint symmetric L0 L17.start L82.start
  constraint symmetric L0 L18.end L72.end
  constraint symmetric L0 L19.end L77.end
  constraint symmetric L0 L20.end L65.end
  constraint symmetric L0 L22.end L84.end
  constraint symmetric L0 L21.end L85.start
  constraint symmetric L0 L25.end L76.end
  constraint symmetric L0 L26.end L67.start
  constraint symmetric L0 L27.end L75.end
  constraint symmetric L0 L28.end L66.start
  constraint symmetric L0 L31.end L70.end
  constraint symmetric L0 L32.end L69.start
  constraint symmetric L0 L33.end L69.end
  constraint symmetric L0 L34.end L74.end
  constraint symmetric L0 L38.end L73.end
  constraint symmetric L0 L39.end L81.end
  constraint symmetric L0 A4 A10
  constraint symmetric L0 A5 A8
  constraint symmetric L0 A6 A11
  constraint symmetric L0 A7 A9
  constraint symmetric L2 L0.start L1.start
  constraint symmetric L2 L9.end L110.end
  constraint symmetric L2 L12.end L99.start
  constraint symmetric L2 L15.end L104.end
  constraint symmetric L2 L16.end L99.end
  constraint symmetric L2 L41.end L95.end
  constraint symmetric L2 L42.end L94.start
  constraint symmetric L2 L61.start L93.end
  constraint symmetric L2 L59.start L106.start
  constraint symmetric L2 L43.start L102.start
  constraint symmetric L2 L43.end L102.end
  constraint symmetric L2 L44.end L103.end
  constraint symmetric L2 L42.start L117.end
  constraint symmetric L2 L41.start L115.start
  constraint symmetric L2 L47.start L91.start
  constraint symmetric L2 L47.end L92.start
  constraint symmetric L2 L48.end L91.end
  constraint symmetric L2 L49.end L93.start
  constraint symmetric L2 L50.end L92.end
  constraint symmetric L2 L51.start L100.start
  constraint symmetric L2 L51.end L101.start
  constraint symmetric L2 L52.end L98.start
  constraint symmetric L2 L53.end L98.end
  constraint symmetric L2 L54.end L95.start
  constraint symmetric L2 L55.start L105.start
  constraint symmetric L2 L55.end L97.start
  constraint symmetric L2 L56.end L96.start
  constraint symmetric L2 L57.end L96.end
  constraint symmetric L2 L58.end L97.end
  constraint symmetric L2 A0 A12
  constraint symmetric L2 A1 A13
  constraint symmetric L2 A2 A14
  constraint symmetric L2 A3 A15
  measures "d294" angle of L7 L8
  measures "d295" angle of L9 L10
  measures "d296" distance of L0.start L11.end
  measures "d297" distance of L0.start L12.end
  measures "d298" distance of L11.end L13.end
  measures "d299" distance of L11.end L14.end
  measures "d300" distance of L12.end L15.end
  measures "d301" distance of L12.end L16.end
  measures "d305" distance of L17.end L23.start
  measures "d306" distance of L23.start L24.end
  measures "d307" distance of L24.end L18.start
  measures "d318" distance of L19.start L19.end
  measures "d319" distance of L19.start L20.end
  measures "d321" distance of L25.start L25.end
  measures "d322" distance of L25.start L26.end
  measures "d324" distance of L31.start L31.end
  measures "d325" distance of L31.start L32.end
  measures "d328" distance of L18.end L38.end
  measures "d333" distance of L42.end L61.start
  measures "d334" distance of L61.start L59.start
  measures "d336" distance of L43.start L43.end
  measures "d337" distance of L43.start L44.end
  measures "d340" distance of L47.start L47.end
  measures "d341" distance of L47.start L48.end
  measures "d344" distance of L51.start L51.end
  measures "d345" distance of L51.start L52.end
  measures "d348" distance of L55.start L55.end
  measures "d349" distance of L55.start L56.end
  measures "d365" diameter of A0
  measures "d367" diameter of A1
  measures "d369" diameter of A2
  measures "d371" diameter of A3
  measures "d373" diameter of A4
  measures "d375" diameter of A5
  measures "d377" diameter of A6
  measures "d379" diameter of A7
sketch "Esboço17" plane through (0, 0, 0) normal (0, 1, 0) x (1, 0, 0)
  line L0 (-16, 63.0977) -> (-16, 51.5)
  line L1 (-16, 51.5) -> (0, 51.5)
  arc A0 (-29.453, 60.7352) -> (29.453, 60.7352) centre (0, 0) ccw
  line L2 (-29.453, 60.7352) -> (-16, 63.0977)
  line L3 (29.453, 60.7352) -> (16, 63.0977)
  line L4 (16, 63.0977) -> (16, 51.5)
  line L5 (16, 51.5) -> (0, 51.5)
  dimension "d351" = 135
  constraint coincident A0.centre origin
  measures "d351" diameter of A0
extrude "Extrusão16" add sketch "Esboço17" along normal blind 4
extrude "Extrusão17" cut sketch "Esboço15" along normal blind 1.5
extrude "Extrusão18" cut 16 faces at (57.8553, 0, 19.686) (32.8739, 0, 32.9101) (44.0815, 0, 44.1177) (19.6522, 0, 58.0544) (-20.5115, 0, 58.0544) (-33.877, 0, 32.9101) (-45.0846, 0, 44.1177) (-57.5446, 0, 19.686) (58.5113, 0, -15.262) (47.8359, 0, -41.0253) (36.3509, 0, -30.7675) (25.5185, 0, -54.9899) (-24.6267, 0, -54.9899) (-48.8389, 0, -41.0253) (-36.0403, 0, -30.7675) (-60.0265, 0, -15.262) along direction (0, 1, 0) blind 10
equation "d306 = ( 24.1 * 2 ) * 1 mm"
equation "d334 = ( 24.1 * 2 ) * 1 mm"
